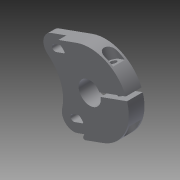
# Autodesk Inventor part: mount_base
Saved by Autodesk Inventor 2015 (Build 190159000, 159)
## iProperties
Created: 2014-11-17
Part Number: mount_base
Material: Generic
Document SubType Name: Modeling
Designer: brent
Density: 1 g/cm^3
Appearance: Default
Mass: 34.4938 g
Surface Area: 117.458 cm^2
Volume: 34.4938 cm^3
Author: brent
Autodesk Inventor part; units mm, degrees
ref_plane "YZ Plane" through (0, 0, 0) normal (1, 0, 0) x (0, 1, 0)
ref_plane "XZ Plane" through (0, 0, 0) normal (0, 1, 0) x (-1, 0, 0)
derived "mount_sketch.ipt"
sketch "Sketch2" plane through (0, 0, 0) normal (0, 0, 1) x (1, 0, 0)
  line L0 (72.439618, -72.294806) -> (-70.244124, 86.171543)
  line L1 (30.373587, -26.37014) -> (-42.626013, -26.37014)
  circle A0 centre (-21.799155, 32.367955) radius 3.96875
  circle A1 centre (-21.799155, 32.367955) radius 9
  circle A2 centre (-82.068234, 4.392394) radius 2.15
  line L2 (-82.068234, 4.392394) -> (-108.233982, 19.067326)
  circle A3 centre (-108.233982, 19.067326) radius 2.15
  line L3 (-87.813642, 24.812734) -> (-102.488574, -1.353014)
  circle A4 centre (-87.813642, 24.812734) radius 2.15
  circle A5 centre (-102.488574, -1.353014) radius 2.15
  line L4 (-95.151108, 11.72986) -> (-21.799155, 32.367955)
  line L5 (-86.578986, -18.737191) -> (-13.227033, 1.900903)
  line L6 (-103.72323, 42.196912) -> (-30.371277, 62.835006)
  circle A6 centre (-95.151108, 11.72986) radius 10.5
  arc A7 (-103.72323, 42.196912) -> (-86.578986, -18.737191) centre (-95.151108, 11.72986) ccw
  circle A8 centre (-21.799155, 32.367955) radius 31.65
  line L7 (-13.662976, 36.215368) -> (8.227399, 42.37438)
  line L8 (-12.850452, 33.327495) -> (9.039922, 39.486508)
  line L9 (-57.877714, 55.095874) -> (-30.371277, 62.835006)
  line L10 (-40.73347, -5.838229) -> (-13.227033, 1.900903)
  arc A9 (-52.432254, 6.081957) -> (-61.644553, 38.824326) centre (-82.733258, 15.223711) ccw
  arc A10 (-57.877714, 55.095874) -> (-61.644553, 38.824326) centre (-55.297952, 45.92688) ccw
  arc A11 (-52.432254, 6.081957) -> (-40.73347, -5.838229) centre (-43.313232, 3.330766) ccw
  line L11 (-55.297952, 45.92688) -> (-49.185289, 47.646721) construction
  line L12 (-54.606576, 43.46959) -> (-48.493913, 45.189431)
  line L13 (-49.876665, 50.104012) -> (-55.989328, 48.384171)
  arc A12 (-55.989328, 48.384171) -> (-54.606576, 43.46959) centre (-55.297952, 45.92688) ccw
  arc A13 (-48.493913, 45.189431) -> (-49.876665, 50.104012) centre (-49.185289, 47.646721) ccw
  line L14 (-43.313232, 3.330766) -> (-37.200569, 5.050607) construction
  line L15 (-42.621855, 0.873475) -> (-36.509193, 2.593316)
  line L16 (-37.891945, 7.507897) -> (-44.004608, 5.788056)
  arc A14 (-44.004608, 5.788056) -> (-42.621855, 0.873475) centre (-43.313232, 3.330766) ccw
  arc A15 (-36.509193, 2.593316) -> (-37.891945, 7.507897) centre (-37.200569, 5.050607) ccw
  circle A16 centre (-52.24162, 46.786801) radius 2.413
  circle A17 centre (-40.2569, 4.190686) radius 2.413
  arc A18 (-37.677138, -4.978308) -> (-42.836662, 13.35968) centre (-40.2569, 4.190686) ccw
  arc A19 (-49.661859, 37.617807) -> (-54.821382, 55.955795) centre (-52.24162, 46.786801) ccw
  arc A20 (-49.661859, 37.617807) -> (-42.836662, 13.35968) centre (-21.799155, 32.367955) ccw
  line L17 (-52.24162, 46.786801) -> (-40.2569, 4.190686)
  point P0 (0, 0)
  point P1 (-91.30538, 45.690762)
  point P2 (-74.161136, -15.243341)
  point P3 (-52.24162, 46.786801)
  point P4 (-40.2569, 4.190686)
sketch "Sketch3" plane through (0, 0, 0) normal (0, 0, 1) x (1, 0, 0)
  arc A0 (-57.877714, 55.095874) -> (-61.644553, 38.824326) centre (-55.297952, 45.92688) ccw
  arc A1 (-52.432254, 6.081957) -> (-61.644553, 38.824326) centre (-82.733258, 15.223711) ccw
  arc A2 (-52.432254, 6.081957) -> (-40.73347, -5.838229) centre (-43.313232, 3.330766) ccw
  line L0 (-40.73347, -5.838229) -> (-13.227033, 1.900903)
  line L1 (-13.662976, 36.215368) -> (8.227399, 42.37438)
  line L2 (-12.850452, 33.327495) -> (9.039922, 39.486508)
  circle A3 centre (-21.799155, 32.367955) radius 9
  line L3 (-57.877714, 55.095874) -> (-30.371277, 62.835006)
  line L4 (-54.606576, 43.46959) -> (-48.493913, 45.189431)
  arc A4 (-48.493913, 45.189431) -> (-49.876665, 50.104012) centre (-49.185289, 47.646721) ccw
  line L5 (-49.876665, 50.104012) -> (-55.989328, 48.384171)
  arc A5 (-55.989328, 48.384171) -> (-54.606576, 43.46959) centre (-55.297952, 45.92688) ccw
  arc A6 (-44.004608, 5.788056) -> (-42.621855, 0.873475) centre (-43.313232, 3.330766) ccw
  line L6 (-42.621855, 0.873475) -> (-36.509193, 2.593316)
  line L7 (-37.891945, 7.507897) -> (-44.004608, 5.788056)
  arc A7 (-36.509193, 2.593316) -> (-37.891945, 7.507897) centre (-37.200569, 5.050607) ccw
  arc A8 (-13.662976, 36.215368) -> (-12.850452, 33.327495) centre (-21.799155, 32.367955) ccw
  arc A9 (-12.850452, 33.327495) -> (-13.662976, 36.215368) centre (-21.799155, 32.367955) ccw
  arc A10 (8.227399, 42.37438) -> (-30.371277, 62.835006) centre (-21.799155, 32.367955) ccw
  arc A11 (9.039922, 39.486508) -> (8.227399, 42.37438) centre (-21.799155, 32.367955) ccw
  arc A12 (-13.227033, 1.900903) -> (9.039922, 39.486508) centre (-21.799155, 32.367955) ccw
  point P0 (0, 0)
  constraints: 10 point on circle, 6 end point, 5 centre point, 2 coincident, 1 concentric
extrude "Extrusion1" add sketch "Sketch3" along normal blind 12.7 contours L3 A10 L1 A3 L2 A12 L0 A2 A1 A0
sketch "Sketch4" plane through (-13.227033, 1.900903, 0) normal (0.2708411, -0.9626241, 0) x (0.9626241, 0.2708411, 0)
  line L0 (0, 0) -> (31.614435, 0)
  line L1 (31.614435, 0) -> (31.614435, 12.7)
  line L2 (0, 12.7) -> (31.614435, 12.7)
  line L3 (0, 0) -> (0, 12.7)
  line L4 (8.87412, 0) -> (31.614435, 0)
  line L5 (31.614435, 0) -> (31.614435, 12.7)
  line L6 (8.87412, 12.7) -> (31.614435, 12.7)
  line L7 (8.87412, 0) -> (8.87412, 12.7)
  line L8 (31.614435, 6.35) -> (20.244277, 6.35) construction
  line L9 (31.614435, 11.1125) -> (20.244277, 11.1125)
  line L10 (20.244277, 1.5875) -> (31.614435, 1.5875)
  arc A0 (31.614435, 1.5875) -> (31.614435, 11.1125) centre (31.614435, 6.35) ccw
  arc A1 (20.244277, 11.1125) -> (20.244277, 1.5875) centre (20.244277, 6.35) ccw
  point P0 (12.217817, 0)
  point P1 (25.929356, 6.35)
  dimension "d3" = 9.525
  dimension "d4" = 22.74032
  dimension "d5" = 11.37016
  constraints: 8 end point, 4 point on circle, 4 tangent, 2 centre point, 2 midpoint, 1 horizontal, 1 parallel
  measures "d3" diameter of A1
  measures "d4" distance between parallel lines of L1 L7
  measures "d5" distance from line of L7 L8.end
extrude "Extrusion2" cut sketch "Sketch4" against normal blind 12.7 contours L10 A1 L9 L1 | L1 A0
ref_plane "Work Plane1" through (-13.256714, 34.771432, 12.7) normal (-0.2708411, 0.9626241, 0) x (0.9626241, 0.2708411, 0)
mirror "Mirror1" about plane through (-13.256714, 34.771432, 12.7) normal (-0.2708411, 0.9626241, 0) of "Extrusion2"
sketch "Sketch5" plane through (-16.666715, 14.126229, 0) normal (0.2708411, -0.9626241, 0) x (0.9626241, 0.2708411, 0)
  line L0 (25.349951, 11.1125) -> (25.349951, 1.5875)
  line L1 (20.244277, 11.1125) -> (25.349951, 11.1125)
  arc A0 (20.244277, 11.1125) -> (20.244277, 1.5875) centre (20.244277, 6.35) ccw
  line L2 (25.349951, 1.5875) -> (20.244277, 1.5875)
  circle A1 centre (20.244277, 6.35) radius 2.5527
  point P0 (12.217817, 0)
  dimension "d8" = 5.1054
  constraints: 1 centre point, 1 coincident
  measures "d8" diameter of A1
extrude "Extrusion3" cut sketch "Sketch5" against normal through all contours A1
sketch "Sketch6" plane through (0, 0, 12.7) normal (0, 0, 1) x (1, 0, 0)
  line L0 (-44.004608, 5.788056) -> (-37.891945, 7.507897)
  arc A0 (-36.509193, 2.593316) -> (-37.891945, 7.507897) centre (-37.200569, 5.050607) ccw
  line L1 (-36.509193, 2.593316) -> (-42.621855, 0.873475)
  arc A1 (-44.004608, 5.788056) -> (-42.621855, 0.873475) centre (-43.313232, 3.330766) ccw
  arc A2 (-55.989328, 48.384171) -> (-54.606576, 43.46959) centre (-55.297952, 45.92688) ccw
  line L2 (-55.989328, 48.384171) -> (-49.876665, 50.104012)
  arc A3 (-48.493913, 45.189431) -> (-49.876665, 50.104012) centre (-49.185289, 47.646721) ccw
  line L3 (-48.493913, 45.189431) -> (-54.606576, 43.46959)
  arc A4 (-57.877714, 55.095874) -> (-61.644553, 38.824326) centre (-55.297952, 45.92688) ccw
  arc A5 (-52.432254, 6.081957) -> (-61.644553, 38.824326) centre (-82.733258, 15.223711) ccw
  arc A6 (-52.432254, 6.081957) -> (-40.73347, -5.838229) centre (-43.313232, 3.330766) ccw
  line L4 (-40.73347, -5.838229) -> (-13.227033, 1.900903)
  arc A7 (-13.227033, 1.900903) -> (9.039922, 39.486508) centre (-21.799155, 32.367955) ccw
  line L5 (9.039922, 39.486508) -> (-12.850452, 33.327495)
  arc A8 (-13.662976, 36.215368) -> (-12.850452, 33.327495) centre (-21.799155, 32.367955) ccw
  line L6 (-13.662976, 36.215368) -> (8.227399, 42.37438)
  arc A9 (8.227399, 42.37438) -> (-30.371277, 62.835006) centre (-21.799155, 32.367955) ccw
  line L7 (-30.371277, 62.835006) -> (-57.877714, 55.095874)
  line L8 (-55.297952, 45.92688) -> (-49.185289, 47.646721) construction
  line L9 (-52.71819, 36.757886) -> (-46.605527, 38.477727)
  line L10 (-51.765051, 56.815716) -> (-57.877714, 55.095874)
  arc A10 (-57.877714, 55.095874) -> (-52.71819, 36.757886) centre (-55.297952, 45.92688) ccw
  arc A11 (-46.605527, 38.477727) -> (-43.590465, 39.938053) centre (-49.185289, 47.646721) ccw
  line L11 (-43.313232, 3.330766) -> (-37.200569, 5.050607) construction
  line L12 (-45.892993, 12.49976) -> (-39.780331, 14.219601)
  line L13 (-34.620807, -4.118387) -> (-40.73347, -5.838229)
  arc A12 (-45.892993, 12.49976) -> (-40.73347, -5.838229) centre (-43.313232, 3.330766) ccw
  arc A13 (-34.620807, -4.118387) -> (-31.417474, 12.619057) centre (-37.200569, 5.050607) ccw
  arc A14 (-37.461305, 14.572038) -> (-39.780331, 14.219601) centre (-37.200569, 5.050607) ccw
  arc A15 (-43.590465, 39.938053) -> (-40.867239, 43.006068) centre (-49.185289, 47.646721) ccw
  arc A16 (-40.033628, 45.006129) -> (-51.765051, 56.815716) centre (-49.185289, 47.646721) ccw
  arc A17 (-31.417474, 12.619057) -> (-32.522664, 13.347765) centre (-37.200569, 5.050607) ccw
  arc A18 (-40.867239, 43.006068) -> (-40.033628, 45.006129) centre (-49.185289, 47.646721) ccw
  arc A19 (-32.522664, 13.347765) -> (-37.461305, 14.572038) centre (-37.200569, 5.050607) ccw
  arc A20 (-40.867239, 43.006068) -> (-32.522664, 13.347765) centre (-21.799155, 32.367955) ccw
  point P0 (0, 0)
  point P1 (-52.24162, 46.786801)
  point P2 (-40.2569, 4.190686)
  constraints: 22 point on circle, 16 end point, 15 tangent, 11 centre point, 3 parallel, 2 midpoint, 1 coincident, 1 point on line
extrude "Extrusion4" cut sketch "Sketch6" against normal blind 6.35 contours L7 A16 A18 A15 A11 L9 A10 A4 | A10 L9 A11 A15 A20 A19 A14 L12 A12 A5 | A12 L12 A14 A19 A17 A13 L4 A6
fillet "Fillet1" radius 1.27 2 edges at (-34.6208, -4.1184, 9.525) (-51.7651, 56.8157, 9.525)
equation "\"d5\" = 0.5 * d4"
body "Solid1"
